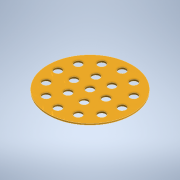
# Autodesk Inventor part: separator_v2
Saved by Autodesk Inventor 2022 (Build 260153000, 153)
## iProperties
Created: 2021-07-24
Part Number: separator_v2
Material: Brass, Soft Yellow, Welded
Document SubType Name: Modeling
Designer: WASHINGTON
Density: 8.5 g/cm^3
Appearance: Weld - Brass
Author: WASHINGTON
Autodesk Inventor part; units mm, degrees
ref_plane "YZ Plane" through (0, 0, 0) normal (1, 0, 0) x (0, 1, 0)
ref_plane "XZ Plane" through (0, 0, 0) normal (0, 1, 0) x (-1, 0, 0)
ref_plane "XY Plane" through (0, 0, 0) normal (0, 0, 1) x (1, 0, 0)
sketch "Sketch1" plane through (0, 0, 0) normal (0, 1, 0) x (-1, 0, 0)
  circle A0 centre (0, 0) radius 55
  line L0 (0, 0) -> (15, 0)
  circle A1 centre (0, 0) radius 8 construction
  line L1 (0, 0) -> (21, 0)
  circle A2 centre (21, 0) radius 8 construction
  line L2 (0, 0) -> (42, 0)
  circle A3 centre (42, 0) radius 8 construction
  circle A4 centre (0, 0) radius 5
  circle A5 centre (21, 0) radius 5
  circle A6 centre (10.5, 18.1865) radius 5
  circle A7 centre (-10.5, 18.1865) radius 5
  circle A8 centre (-21, 0) radius 5
  circle A9 centre (-10.5, -18.1865) radius 5
  circle A10 centre (10.5, -18.1865) radius 5
  circle A11 centre (42, 0) radius 5
  circle A12 centre (36.3731, 21) radius 5
  circle A13 centre (21, 36.3731) radius 5
  circle A14 centre (0, 42) radius 5
  circle A15 centre (-21, 36.3731) radius 5
  circle A16 centre (-36.3731, 21) radius 5
  circle A17 centre (-42, 0) radius 5
  circle A18 centre (-36.3731, -21) radius 5
  circle A19 centre (-21, -36.3731) radius 5
  circle A20 centre (0, -42) radius 5
  circle A21 centre (21, -36.3731) radius 5
  circle A22 centre (36.3731, -21) radius 5
  dimension "d0" = 110
  dimension "d4" = 15
  dimension "d6" = 16
  dimension "d7" = 21
  dimension "d8" = 16
  dimension "d14" = 42
  dimension "d15" = 16
  dimension "d20" = 10
  dimension "d21" = 10
  dimension "d24" = 360
  dimension "d26" = 10
  dimension "d29" = 360
  constraints: 23 centre point, 8 coincident, 6 end point, 2 horizontal, 1 point on line, 38 other
  measures "d0" diameter of A0
  measures "d4" distance of L0.start L0.end
  measures "d6" diameter of A1
  measures "d7" distance of L1.start L1.end
  measures "d8" diameter of A2
  measures "d14" distance of L1.start L2.end
  measures "d15" diameter of A3
  measures "d20" diameter of A4
  measures "d21" diameter of A5
  measures "d26" diameter of A11
extrude "Extrusion1" add sketch "Sketch1" along normal blind 2
body "Solid1"
